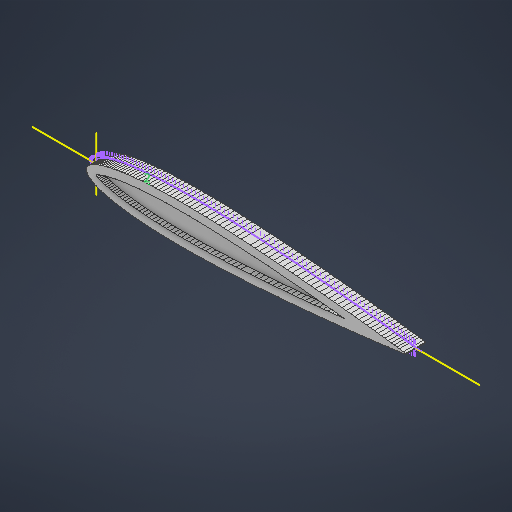
# Autodesk Inventor part: Profil NACA 0012
Saved by Autodesk Inventor 2026 (Build 300175050, 175E)
## iProperties
Created: 2026-02-21
Part Number: Profil NACA 0012
Material: Všeobecné
Document SubType Name: Modeling
Designer: marti
Density: 1 g/cm^3
Appearance: Výchozí
Author: marti
Autodesk Inventor part; units mm, degrees
ref_plane "YZ Plane" through (0, 0, 0) normal (1, 0, 0) x (0, 1, 0)
ref_plane "XZ Plane" through (0, 0, 0) normal (0, 1, 0) x (-1, 0, 0)
ref_plane "XY Plane" through (0, 0, 0) normal (0, 0, 1) x (1, 0, 0)
sketch "Náčrt1" plane through (0, 0, 0) normal (0, 0, 1) x (1, 0, 0)
  line L0 (0, 0) -> (0.0153, -0.1956)
  line L1 (0.0153, -0.1956) -> (0.0608, -0.3883)
  line L2 (0.0608, -0.3883) -> (0.1363, -0.578)
  line L3 (0.1363, -0.578) -> (0.2416, -0.7647)
  line L4 (0.2416, -0.7647) -> (0.3761, -0.9484)
  line L5 (0.3761, -0.9484) -> (0.5397, -1.129)
  line L6 (0.5397, -1.129) -> (0.732, -1.3065)
  line L7 (0.732, -1.3065) -> (0.9527, -1.4808)
  line L8 (0.9527, -1.4808) -> (1.2014, -1.6519)
  line L9 (1.2014, -1.6519) -> (1.4779, -1.8196)
  line L10 (1.4779, -1.8196) -> (1.7818, -1.9839)
  line L11 (1.7818, -1.9839) -> (2.1127, -2.1447)
  line L12 (2.1127, -2.1447) -> (2.4703, -2.3018)
  line L13 (2.4703, -2.3018) -> (2.8543, -2.4552)
  line L14 (2.8543, -2.4552) -> (3.2643, -2.6048)
  line L15 (3.2643, -2.6048) -> (3.7, -2.7504)
  line L16 (3.7, -2.7504) -> (4.1611, -2.8918)
  line L17 (4.1611, -2.8918) -> (4.6471, -3.0291)
  line L18 (4.6471, -3.0291) -> (5.1577, -3.162)
  line L19 (5.1577, -3.162) -> (5.6926, -3.2905)
  line L20 (5.6926, -3.2905) -> (6.2513, -3.4144)
  line L21 (6.2513, -3.4144) -> (6.8335, -3.5336)
  line L22 (6.8335, -3.5336) -> (7.4389, -3.648)
  line L23 (7.4389, -3.648) -> (8.0671, -3.7575)
  line L24 (8.0671, -3.7575) -> (8.7176, -3.8619)
  line L25 (8.7176, -3.8619) -> (9.3901, -3.9612)
  line L26 (9.3901, -3.9612) -> (10.0843, -4.0553)
  line L27 (10.0843, -4.0553) -> (10.7996, -4.1441)
  line L28 (10.7996, -4.1441) -> (11.5357, -4.2274)
  line L29 (11.5357, -4.2274) -> (12.2923, -4.3053)
  line L30 (12.2923, -4.3053) -> (13.0688, -4.3777)
  line L31 (13.0688, -4.3777) -> (13.865, -4.4444)
  line L32 (13.865, -4.4444) -> (14.6803, -4.5055)
  line L33 (14.6803, -4.5055) -> (15.5143, -4.5609)
  line L34 (15.5143, -4.5609) -> (16.3667, -4.6106)
  line L35 (16.3667, -4.6106) -> (17.2369, -4.6545)
  line L36 (17.2369, -4.6545) -> (18.1246, -4.6927)
  line L37 (18.1246, -4.6927) -> (19.0293, -4.7251)
  line L38 (19.0293, -4.7251) -> (19.9505, -4.7517)
  line L39 (19.9505, -4.7517) -> (20.8878, -4.7726)
  line L40 (20.8878, -4.7726) -> (21.8407, -4.7879)
  line L41 (21.8407, -4.7879) -> (22.8088, -4.7974)
  line L42 (22.8088, -4.7974) -> (23.7915, -4.8013)
  line L43 (23.7915, -4.8013) -> (24.7885, -4.7996)
  line L44 (24.7885, -4.7996) -> (25.7991, -4.7924)
  line L45 (25.7991, -4.7924) -> (26.8229, -4.7797)
  line L46 (26.8229, -4.7797) -> (27.8593, -4.7617)
  line L47 (27.8593, -4.7617) -> (28.908, -4.7384)
  line L48 (28.908, -4.7384) -> (29.9682, -4.71)
  line L49 (29.9682, -4.71) -> (31.0396, -4.6764)
  line L50 (31.0396, -4.6764) -> (32.1215, -4.6379)
  line L51 (32.1215, -4.6379) -> (33.2133, -4.5945)
  line L52 (33.2133, -4.5945) -> (34.3147, -4.5463)
  line L53 (34.3147, -4.5463) -> (35.4248, -4.4935)
  line L54 (35.4248, -4.4935) -> (36.5432, -4.4363)
  line L55 (36.5432, -4.4363) -> (37.6693, -4.3747)
  line L56 (37.6693, -4.3747) -> (38.802, -4.3088)
  line L57 (38.802, -4.3088) -> (41.0871, -4.165)
  line L58 (41.0871, -4.165) -> (42.2375, -4.0874)
  line L59 (42.2375, -4.0874) -> (43.3923, -4.006)
  line L60 (43.3923, -4.006) -> (44.5509, -3.9212)
  line L61 (44.5509, -3.9212) -> (45.7124, -3.833)
  line L62 (45.7124, -3.833) -> (46.8763, -3.7417)
  line L63 (46.8763, -3.7417) -> (48.0418, -3.6473)
  line L64 (48.0418, -3.6473) -> (49.208, -3.5499)
  line L65 (49.208, -3.5499) -> (50.3742, -3.4499)
  line L66 (50.3742, -3.4499) -> (51.5396, -3.3473)
  line L67 (51.5396, -3.3473) -> (52.7034, -3.2422)
  line L68 (52.7034, -3.2422) -> (53.8647, -3.1348)
  line L69 (53.8647, -3.1348) -> (55.0224, -3.0254)
  line L70 (55.0224, -3.0254) -> (56.1759, -2.914)
  line L71 (56.1759, -2.914) -> (57.324, -2.8008)
  line L72 (57.324, -2.8008) -> (58.4658, -2.686)
  line L73 (58.4658, -2.686) -> (59.6001, -2.5697)
  line L74 (59.6001, -2.5697) -> (60.726, -2.4522)
  line L75 (60.726, -2.4522) -> (61.8422, -2.3336)
  line L76 (61.8422, -2.3336) -> (62.9476, -2.2141)
  line L77 (62.9476, -2.2141) -> (64.041, -2.094)
  line L78 (64.041, -2.094) -> (65.1209, -1.9733)
  line L79 (65.1209, -1.9733) -> (66.186, -1.8524)
  line L80 (66.186, -1.8524) -> (67.2348, -1.7315)
  line L81 (67.2348, -1.7315) -> (68.2656, -1.6108)
  line L82 (68.2656, -1.6108) -> (69.2769, -1.4906)
  line L83 (69.2769, -1.4906) -> (70.2666, -1.3713)
  line L84 (70.2666, -1.3713) -> (71.233, -1.2532)
  line L85 (71.233, -1.2532) -> (72.1737, -1.1365)
  line L86 (72.1737, -1.1365) -> (73.0864, -1.0218)
  line L87 (73.0864, -1.0218) -> (73.9685, -0.9095)
  line L88 (73.9685, -0.9095) -> (74.817, -0.8001)
  line L89 (74.817, -0.8001) -> (75.6285, -0.6942)
  line L90 (75.6285, -0.6942) -> (76.3992, -0.5924)
  line L91 (76.3992, -0.5924) -> (77.1245, -0.4955)
  line L92 (77.1245, -0.4955) -> (77.7988, -0.4045)
  line L93 (77.7988, -0.4045) -> (78.4151, -0.3205)
  line L94 (78.4151, -0.3205) -> (78.9642, -0.245)
  line L95 (78.9642, -0.245) -> (79.4327, -0.1806)
  line L96 (79.4327, -0.1806) -> (79.7982, -0.1291)
  line L97 (79.7982, -0.1291) -> (80, -0.1006)
  line L98 (0, 6.7218) -> (0, -6.7218) projected
  line L99 (-16, 0) -> (96, 0) projected
  line L100 (0, 0) -> (0.0153, 0.1956)
  line L101 (0.0153, 0.1956) -> (0.0608, 0.3883)
  line L102 (0.0608, 0.3883) -> (0.1363, 0.578)
  line L103 (0.1363, 0.578) -> (0.2416, 0.7647)
  line L104 (0.2416, 0.7647) -> (0.3761, 0.9484)
  line L105 (0.3761, 0.9484) -> (0.5397, 1.129)
  line L106 (0.5397, 1.129) -> (0.732, 1.3065)
  line L107 (0.732, 1.3065) -> (0.9527, 1.4808)
  line L108 (0.9527, 1.4808) -> (1.2014, 1.6519)
  line L109 (1.2014, 1.6519) -> (1.4779, 1.8196)
  line L110 (1.4779, 1.8196) -> (1.7818, 1.9839)
  line L111 (1.7818, 1.9839) -> (2.1127, 2.1447)
  line L112 (2.1127, 2.1447) -> (2.4703, 2.3018)
  line L113 (2.4703, 2.3018) -> (2.8543, 2.4552)
  line L114 (2.8543, 2.4552) -> (3.2643, 2.6048)
  line L115 (3.2643, 2.6048) -> (3.7, 2.7504)
  line L116 (3.7, 2.7504) -> (4.1611, 2.8918)
  line L117 (4.1611, 2.8918) -> (4.6471, 3.0291)
  line L118 (4.6471, 3.0291) -> (5.1577, 3.162)
  line L119 (5.1577, 3.162) -> (5.6926, 3.2905)
  line L120 (5.6926, 3.2905) -> (6.2513, 3.4144)
  line L121 (6.2513, 3.4144) -> (6.8335, 3.5336)
  line L122 (6.8335, 3.5336) -> (7.4389, 3.648)
  line L123 (7.4389, 3.648) -> (8.0671, 3.7575)
  line L124 (8.0671, 3.7575) -> (8.7176, 3.8619)
  line L125 (8.7176, 3.8619) -> (9.3901, 3.9612)
  line L126 (9.3901, 3.9612) -> (10.0843, 4.0553)
  line L127 (10.0843, 4.0553) -> (10.7996, 4.1441)
  line L128 (10.7996, 4.1441) -> (11.5357, 4.2274)
  line L129 (11.5357, 4.2274) -> (12.2923, 4.3053)
  line L130 (12.2923, 4.3053) -> (13.0688, 4.3777)
  line L131 (13.0688, 4.3777) -> (13.865, 4.4444)
  line L132 (13.865, 4.4444) -> (14.6803, 4.5055)
  line L133 (14.6803, 4.5055) -> (15.5143, 4.5609)
  line L134 (15.5143, 4.5609) -> (16.3667, 4.6106)
  line L135 (16.3667, 4.6106) -> (17.2369, 4.6545)
  line L136 (17.2369, 4.6545) -> (18.1246, 4.6927)
  line L137 (18.1246, 4.6927) -> (19.0293, 4.7251)
  line L138 (19.0293, 4.7251) -> (19.9505, 4.7517)
  line L139 (19.9505, 4.7517) -> (20.8878, 4.7726)
  line L140 (20.8878, 4.7726) -> (21.8407, 4.7879)
  line L141 (21.8407, 4.7879) -> (22.8088, 4.7974)
  line L142 (22.8088, 4.7974) -> (23.7915, 4.8013)
  line L143 (23.7915, 4.8013) -> (24.7884, 4.7996)
  line L144 (24.7884, 4.7996) -> (25.7991, 4.7924)
  line L145 (25.7991, 4.7924) -> (26.8228, 4.7797)
  line L146 (26.8228, 4.7797) -> (27.8593, 4.7617)
  line L147 (27.8593, 4.7617) -> (28.9079, 4.7384)
  line L148 (28.9079, 4.7384) -> (29.9682, 4.71)
  line L149 (29.9682, 4.71) -> (31.0395, 4.6764)
  line L150 (31.0395, 4.6764) -> (32.1214, 4.6379)
  line L151 (32.1214, 4.6379) -> (33.2133, 4.5945)
  line L152 (33.2133, 4.5945) -> (34.3146, 4.5463)
  line L153 (34.3146, 4.5463) -> (35.4248, 4.4935)
  line L154 (35.4248, 4.4935) -> (36.5432, 4.4363)
  line L155 (36.5432, 4.4363) -> (37.6693, 4.3747)
  line L156 (37.6693, 4.3747) -> (38.8027, 4.3088)
  line L157 (38.8027, 4.3088) -> (41.0871, 4.165)
  line L158 (41.0871, 4.165) -> (42.2375, 4.0874)
  line L159 (42.2375, 4.0874) -> (43.3923, 4.006)
  line L160 (43.3923, 4.006) -> (44.5508, 3.9212)
  line L161 (44.5508, 3.9212) -> (45.7124, 3.833)
  line L162 (45.7124, 3.833) -> (46.8763, 3.7417)
  line L163 (46.8763, 3.7417) -> (48.0417, 3.6473)
  line L164 (48.0417, 3.6473) -> (49.2079, 3.55)
  line L165 (49.2079, 3.55) -> (50.3742, 3.4499)
  line L166 (50.3742, 3.4499) -> (51.5396, 3.3473)
  line L167 (51.5396, 3.3473) -> (52.7033, 3.2422)
  line L168 (52.7033, 3.2422) -> (53.8645, 3.1349)
  line L169 (53.8645, 3.1349) -> (55.0224, 3.0254)
  line L170 (55.0224, 3.0254) -> (56.1757, 2.914)
  line L171 (56.1757, 2.914) -> (57.3238, 2.8008)
  line L172 (57.3238, 2.8008) -> (58.4655, 2.686)
  line L173 (58.4655, 2.686) -> (59.6, 2.5698)
  line L174 (59.6, 2.5698) -> (60.7259, 2.4522)
  line L175 (60.7259, 2.4522) -> (61.8422, 2.3336)
  line L176 (61.8422, 2.3336) -> (62.9477, 2.2141)
  line L177 (62.9477, 2.2141) -> (64.041, 2.094)
  line L178 (64.041, 2.094) -> (65.1209, 1.9733)
  line L179 (65.1209, 1.9733) -> (66.186, 1.8524)
  line L180 (66.186, 1.8524) -> (67.2348, 1.7315)
  line L181 (67.2348, 1.7315) -> (68.2656, 1.6108)
  line L182 (68.2656, 1.6108) -> (69.2769, 1.4906)
  line L183 (69.2769, 1.4906) -> (70.2666, 1.3713)
  line L184 (70.2666, 1.3713) -> (71.233, 1.2532)
  line L185 (71.233, 1.2532) -> (72.1737, 1.1365)
  line L186 (72.1737, 1.1365) -> (73.0864, 1.0218)
  line L187 (73.0864, 1.0218) -> (73.9685, 0.9095)
  line L188 (73.9685, 0.9095) -> (74.817, 0.8001)
  line L189 (74.817, 0.8001) -> (75.6285, 0.6942)
  line L190 (75.6285, 0.6942) -> (76.3992, 0.5924)
  line L191 (76.3992, 0.5924) -> (77.1245, 0.4955)
  line L192 (77.1245, 0.4955) -> (77.7988, 0.4045)
  line L193 (77.7988, 0.4045) -> (78.4151, 0.3205)
  line L194 (78.4151, 0.3205) -> (78.9642, 0.245)
  line L195 (78.9642, 0.245) -> (79.4327, 0.1806)
  line L196 (79.4327, 0.1806) -> (79.7982, 0.1291)
  line L197 (79.7982, 0.1291) -> (80, 0.1006)
  line L198 (80, 0.1006) -> (80, -0.1006)
  line L199 (13.2451, 2.3854) -> (12.4875, 2.3148)
  line L200 (12.4875, 2.3148) -> (11.7507, 2.239)
  line L201 (11.7507, 2.239) -> (11.0353, 2.158)
  line L202 (11.0353, 2.158) -> (10.3417, 2.0719)
  line L203 (10.3417, 2.0719) -> (9.6705, 1.9809)
  line L204 (9.6705, 1.9809) -> (9.0222, 1.8852)
  line L205 (9.0222, 1.8852) -> (8.3973, 1.7849)
  line L206 (8.3973, 1.7849) -> (7.7963, 1.6802)
  line L207 (7.7963, 1.6802) -> (7.2198, 1.5712)
  line L208 (7.2198, 1.5712) -> (6.6684, 1.4583)
  line L209 (6.6684, 1.4583) -> (6.1426, 1.3418)
  line L210 (6.1426, 1.3418) -> (5.6433, 1.2218)
  line L211 (5.6433, 1.2218) -> (5.1709, 1.0988)
  line L212 (5.1709, 1.0988) -> (4.7263, 0.9733)
  line L213 (4.7263, 0.9733) -> (4.3104, 0.8456)
  line L214 (4.3104, 0.8456) -> (3.924, 0.7165)
  line L215 (3.924, 0.7165) -> (3.5681, 0.5867)
  line L216 (3.5681, 0.5867) -> (3.2438, 0.4571)
  line L217 (3.2438, 0.4571) -> (2.9523, 0.329)
  line L218 (2.9523, 0.329) -> (2.6948, 0.204)
  line L219 (2.6948, 0.204) -> (2.4729, 0.0839)
  line L220 (2.4729, 0.0839) -> (2.3345, 0)
  line L221 (2.3345, 0) -> (2.4729, -0.0839)
  line L222 (2.4729, -0.0839) -> (2.6948, -0.204)
  line L223 (2.6948, -0.204) -> (2.9523, -0.329)
  line L224 (2.9523, -0.329) -> (3.2438, -0.4571)
  line L225 (3.2438, -0.4571) -> (3.5681, -0.5867)
  line L226 (3.5681, -0.5867) -> (3.924, -0.7165)
  line L227 (3.924, -0.7165) -> (4.3104, -0.8456)
  line L228 (4.3104, -0.8456) -> (4.7263, -0.9733)
  line L229 (4.7263, -0.9733) -> (5.1709, -1.0988)
  line L230 (5.1709, -1.0988) -> (5.6433, -1.2218)
  line L231 (5.6433, -1.2218) -> (6.1426, -1.3418)
  line L232 (6.1426, -1.3418) -> (6.6684, -1.4583)
  line L233 (6.6684, -1.4583) -> (7.2198, -1.5712)
  line L234 (7.2198, -1.5712) -> (7.7963, -1.6802)
  line L235 (7.7963, -1.6802) -> (8.3973, -1.7849)
  line L236 (8.3973, -1.7849) -> (9.0222, -1.8852)
  line L237 (9.0222, -1.8852) -> (9.6705, -1.9809)
  line L238 (9.6705, -1.9809) -> (10.3417, -2.0719)
  line L239 (10.3417, -2.0719) -> (11.0353, -2.158)
  line L240 (11.0353, -2.158) -> (11.7507, -2.239)
  line L241 (11.7507, -2.239) -> (12.4875, -2.3148)
  line L242 (12.4875, -2.3148) -> (13.2451, -2.3854)
  line L243 (13.2451, -2.3854) -> (14.0232, -2.4507)
  line L244 (14.0232, -2.4507) -> (14.8213, -2.5105)
  line L245 (14.8213, -2.5105) -> (15.6388, -2.5648)
  line L246 (15.6388, -2.5648) -> (16.4753, -2.6135)
  line L247 (16.4753, -2.6135) -> (17.3303, -2.6567)
  line L248 (17.3303, -2.6567) -> (18.2034, -2.6942)
  line L249 (18.2034, -2.6942) -> (19.094, -2.7261)
  line L250 (19.094, -2.7261) -> (20.0017, -2.7524)
  line L251 (20.0017, -2.7524) -> (20.9261, -2.773)
  line L252 (20.9261, -2.773) -> (21.8665, -2.788)
  line L253 (21.8665, -2.788) -> (22.8226, -2.7974)
  line L254 (22.8226, -2.7974) -> (23.7938, -2.8013)
  line L255 (23.7938, -2.8013) -> (24.7796, -2.7996)
  line L256 (24.7796, -2.7996) -> (25.7796, -2.7925)
  line L257 (25.7796, -2.7925) -> (26.7931, -2.78)
  line L258 (26.7931, -2.78) -> (27.8197, -2.7621)
  line L259 (27.8197, -2.7621) -> (28.8589, -2.739)
  line L260 (28.8589, -2.739) -> (29.91, -2.7108)
  line L261 (29.91, -2.7108) -> (30.9727, -2.6775)
  line L262 (30.9727, -2.6775) -> (32.0461, -2.6393)
  line L263 (32.0461, -2.6393) -> (33.1299, -2.5962)
  line L264 (33.1299, -2.5962) -> (34.2235, -2.5484)
  line L265 (34.2235, -2.5484) -> (35.3262, -2.496)
  line L266 (35.3262, -2.496) -> (36.4374, -2.4391)
  line L267 (36.4374, -2.4391) -> (37.5566, -2.3778)
  line L268 (37.5566, -2.3778) -> (38.6812, -2.3125)
  line L269 (38.6812, -2.3125) -> (40.957, -2.1692)
  line L270 (40.957, -2.1692) -> (42.0999, -2.0921)
  line L271 (42.0999, -2.0921) -> (43.249, -2.0112)
  line L272 (43.249, -2.0112) -> (44.4022, -1.9267)
  line L273 (44.4022, -1.9267) -> (45.5585, -1.839)
  line L274 (45.5585, -1.839) -> (46.7173, -1.748)
  line L275 (46.7173, -1.748) -> (47.8779, -1.654)
  line L276 (47.8779, -1.654) -> (49.0394, -1.5571)
  line L277 (49.0394, -1.5571) -> (50.201, -1.4574)
  line L278 (50.201, -1.4574) -> (51.362, -1.3552)
  line L279 (51.362, -1.3552) -> (52.5214, -1.2505)
  line L280 (52.5214, -1.2505) -> (53.6785, -1.1435)
  line L281 (53.6785, -1.1435) -> (54.8322, -1.0345)
  line L282 (54.8322, -1.0345) -> (55.9816, -0.9234)
  line L283 (55.9816, -0.9234) -> (57.1258, -0.8106)
  line L284 (57.1258, -0.8106) -> (58.2638, -0.6962)
  line L285 (58.2638, -0.6962) -> (59.3944, -0.5804)
  line L286 (59.3944, -0.5804) -> (60.5165, -0.4632)
  line L287 (60.5165, -0.4632) -> (61.6291, -0.345)
  line L288 (61.6291, -0.345) -> (62.7308, -0.2259)
  line L289 (62.7308, -0.2259) -> (63.8207, -0.1061)
  line L290 (63.8207, -0.1061) -> (64.7705, 0)
  line L291 (64.7705, 0) -> (63.8207, 0.1061)
  line L292 (63.8207, 0.1061) -> (62.7309, 0.2259)
  line L293 (62.7309, 0.2259) -> (61.6291, 0.345)
  line L294 (61.6291, 0.345) -> (60.5164, 0.4632)
  line L295 (60.5164, 0.4632) -> (59.3942, 0.5804)
  line L296 (59.3942, 0.5804) -> (58.2636, 0.6962)
  line L297 (58.2636, 0.6962) -> (57.1257, 0.8107)
  line L298 (57.1257, 0.8107) -> (55.9815, 0.9235)
  line L299 (55.9815, 0.9235) -> (54.8321, 1.0345)
  line L300 (54.8321, 1.0345) -> (53.6784, 1.1435)
  line L301 (53.6784, 1.1435) -> (52.5214, 1.2505)
  line L302 (52.5214, 1.2505) -> (51.362, 1.3552)
  line L303 (51.362, 1.3552) -> (50.201, 1.4574)
  line L304 (50.201, 1.4574) -> (49.0393, 1.5571)
  line L305 (49.0393, 1.5571) -> (47.8778, 1.654)
  line L306 (47.8778, 1.654) -> (46.7173, 1.748)
  line L307 (46.7173, 1.748) -> (45.5585, 1.839)
  line L308 (45.5585, 1.839) -> (44.4021, 1.9268)
  line L309 (44.4021, 1.9268) -> (43.2491, 2.0112)
  line L310 (43.2491, 2.0112) -> (42.0999, 2.0921)
  line L311 (42.0999, 2.0921) -> (40.9569, 2.1693)
  line L312 (40.9569, 2.1693) -> (38.6819, 2.3124)
  line L313 (38.6819, 2.3124) -> (37.5566, 2.3778)
  line L314 (37.5566, 2.3778) -> (36.4374, 2.4391)
  line L315 (36.4374, 2.4391) -> (35.3262, 2.496)
  line L316 (35.3262, 2.496) -> (34.2235, 2.5484)
  line L317 (34.2235, 2.5484) -> (33.1299, 2.5962)
  line L318 (33.1299, 2.5962) -> (32.0461, 2.6393)
  line L319 (32.0461, 2.6393) -> (30.9726, 2.6775)
  line L320 (30.9726, 2.6775) -> (29.91, 2.7108)
  line L321 (29.91, 2.7108) -> (28.8589, 2.739)
  line L322 (28.8589, 2.739) -> (27.8197, 2.7621)
  line L323 (27.8197, 2.7621) -> (26.7931, 2.78)
  line L324 (26.7931, 2.78) -> (25.7796, 2.7925)
  line L325 (25.7796, 2.7925) -> (24.7796, 2.7996)
  line L326 (24.7796, 2.7996) -> (23.7938, 2.8013)
  line L327 (23.7938, 2.8013) -> (22.8226, 2.7974)
  line L328 (22.8226, 2.7974) -> (21.8665, 2.788)
  line L329 (21.8665, 2.788) -> (20.9261, 2.773)
  line L330 (20.9261, 2.773) -> (20.0017, 2.7524)
  line L331 (20.0017, 2.7524) -> (19.094, 2.7261)
  line L332 (19.094, 2.7261) -> (18.2034, 2.6942)
  line L333 (18.2034, 2.6942) -> (17.3303, 2.6567)
  line L334 (17.3303, 2.6567) -> (16.4753, 2.6135)
  line L335 (16.4753, 2.6135) -> (15.6388, 2.5648)
  line L336 (15.6388, 2.5648) -> (14.8213, 2.5105)
  line L337 (14.8213, 2.5105) -> (14.0232, 2.4507)
  line L338 (14.0232, 2.4507) -> (13.2451, 2.3854)
  point P0 (0, 0)
  point P1 (39.9419, -4.2389)
  point P2 (39.9419, 4.2389)
  dimension "d0" = 2
  constraints: 674 end point, 2 collinear, 1 vertical, 139 other
  measures "d0" distance between parallel lines of L130 L199
extrude "Vysunutí1" add sketch "Náčrt1" along normal mid plane 5 contours L99 L221 L222 L223 L224 L225 L226 L227 L228 L229 L230 L231 L232 L233 L234 L235 L236 L237 L238 L239 L240 L241 L242 L243 L244 L245 L246 L247 L248 L249 L250 L251 L252 L253 L254 L255 L256 L257 L258 L259 L260 L261 L262 L263 L264 L265 L266 L267 L268 L269 L270 L271 L272 L273 L274 L275 L276 L277 L278 L279 L280 L281 L282 L283 L284 L285 L286 L287 L288 L289 L290 L198 L97 L96 L95 L94 L93 L92 L91 L90 L89 L88 L87 L86 L85 L84 L83 L82 L81 L80 L79 L78 L77 L76 L75 L74 L73 L72 L71 L70 L69 L68 L67 L66 L65 L64 L63 L62 L61 L60 L59 L58 L57 L56 L55 L54 L53 L52 L51 L50 L49 L48 L47 L46 L45 L44 L43 L42 L41 L40 L39 L38 L37 L36 L35 L34 L33 L32 L31 L30 L29 L28 L27 L26 L25 L24 L23 L22 L21 L20 L19 L18 L17 L16 L15 L14 L13 L12 L11 L10 L9 L8 L7 L6 L5 L4 L3 L2 L1 L0 | L100 L101 L102 L103 L104 L105 L106 L107 L108 L109 L110 L111 L112 L113 L114 L115 L116 L117 L118 L119 L120 L121 L122 L123 L124 L125 L126 L127 L128 L129 L130 L131 L132 L133 L134 L135 L136 L137 L138 L139 L140 L141 L142 L143 L144 L145 L146 L147 L148 L149 L150 L151 L152 L153 L154 L155 L156 L157 L158 L159 L160 L161 L162 L163 L164 L165 L166 L167 L168 L169 L170 L171 L172 L173 L174 L175 L176 L177 L178 L179 L180 L181 L182 L183 L184 L185 L186 L187 L188 L189 L190 L191 L192 L193 L194 L195 L196 L197 L198 L99 L291 L292 L293 L294 L295 L296 L297 L298 L299 L300 L301 L302 L303 L304 L305 L306 L307 L308 L309 L310 L311 L312 L313 L314 L315 L316 L317 L318 L319 L320 L321 L322 L323 L324 L325 L326 L327 L328 L329 L330 L331 L332 L333 L334 L335 L336 L337 L338 L199 L200 L201 L202 L203 L204 L205 L206 L207 L208 L209 L210 L211 L212 L213 L214 L215 L216 L217 L218 L219 L220
extrude "Vysunutí2" add sketch "Náčrt1" along normal mid plane 2 contours L220 L219 L218 L217 L216 L215 L214 L213 L212 L211 L210 L209 L208 L207 L206 L205 L204 L203 L202 L201 L200 L199 L338 L337 L336 L335 L334 L333 L332 L331 L330 L329 L328 L327 L326 L325 L324 L323 L322 L321 L320 L319 L318 L317 L316 L315 L314 L313 L312 L311 L310 L309 L308 L307 L306 L305 L304 L303 L302 L301 L300 L299 L298 L297 L296 L295 L294 L293 L292 L291 L99 | L99 L290 L289 L288 L287 L286 L285 L284 L283 L282 L281 L280 L279 L278 L277 L276 L275 L274 L273 L272 L271 L270 L269 L268 L267 L266 L265 L264 L263 L262 L261 L260 L259 L258 L257 L256 L255 L254 L253 L252 L251 L250 L249 L248 L247 L246 L245 L244 L243 L242 L241 L240 L239 L238 L237 L236 L235 L234 L233 L232 L231 L230 L229 L228 L227 L226 L225 L224 L223 L222 L221
